Autodesk Fusion 360 part; units mm, degrees
(part 5 of 6)
  spline S1504 degree 3 poles (-29.6521, 8.8842) (-29.6849, 8.8897) (-29.7178, 8.8951) (-29.7517, 8.9007) knots 0 0 0 0 1 1 1 1
  spline S1505 degree 3 poles (-29.7517, 8.9007) (-30.0899, 8.9662) (-30.2987, 9.1721) (-30.5435, 9.4009) knots 0 0 0 0 1 1 1 1
  spline S1506 degree 3 poles (-30.5435, 9.4009) (-30.5714, 9.4268) (-30.5992, 9.4527) (-30.628, 9.4794) knots 0 0 0 0 1 1 1 1
  spline S1507 degree 3 poles (-30.628, 9.4794) (-30.6858, 9.5332) (-30.7436, 9.587) (-30.8013, 9.6409) knots 0 0 0 0 1 1 1 1
  spline S1508 degree 3 poles (-30.8013, 9.6409) (-30.8812, 9.7151) (-30.9615, 9.7888) (-31.0421, 9.8622) knots 0 0 0 0 1 1 1 1
  spline S1509 degree 3 poles (-31.0421, 9.8622) (-31.5525, 10.3296) (-31.9981, 10.8199) (-32.3801, 11.398) knots 0 0 0 0 1 1 1 1
  spline S1510 degree 3 poles (-32.3801, 11.398) (-32.528, 11.3037) (-32.625, 11.1724) (-32.732, 11.0364) knots 0 0 0 0 1 1 1 1
  spline S1511 degree 3 poles (-32.732, 11.0364) (-33.557, 10.0137) (-34.574, 9.1658) (-35.5651, 8.3103) knots 0 0 0 0 1 1 1 1
  spline S1512 degree 3 poles (-35.5651, 8.3103) (-36.1522, 7.8032) (-36.7179, 7.2786) (-37.2683, 6.7319) knots 0 0 0 0 1 1 1 1
  spline S1513 degree 3 poles (-37.2683, 6.7319) (-37.3268, 6.6738) (-37.3856, 6.6161) (-37.4451, 6.559) knots 0 0 0 0 1 1 1 1
  spline S1514 degree 3 poles (-37.4451, 6.559) (-37.6128, 6.3958) (-37.67, 6.2769) (-37.6736, 6.0447) knots 0 0 0 0 1 1 1 1
  spline S1515 degree 3 poles (-37.6736, 6.0447) (-37.6346, 5.5351) (-37.3928, 5.1499) (-37.0124, 4.8179) knots 0 0 0 0 1 1 1 1
  spline S1516 degree 3 poles (-37.0124, 4.8179) (-36.5513, 4.4276) (-36.5513, 4.4276) (-36.3386, 4.4) knots 0 0 0 0 1 1 1 1
  spline S1517 degree 3 poles (-36.3386, 4.4) (-36.3018, 4.395) (-36.265, 4.3899) (-36.227, 4.3848) knots 0 0 0 0 1 1 1 1
  spline S1518 degree 3 poles (-36.227, 4.3848) (-36.168, 4.377) (-36.168, 4.377) (-36.1079, 4.369) knots 0 0 0 0 1 1 1 1
  spline S1519 degree 3 poles (-36.1079, 4.369) (-35.784, 4.324) (-35.4699, 4.2678) (-35.153, 4.1868) knots 0 0 0 0 1 1 1 1
  spline S1520 degree 3 poles (-35.153, 4.1868) (-34.7861, 4.0991) (-34.7861, 4.0991) (-34.5906, 4.1538) knots 0 0 0 0 1 1 1 1
  spline S1521 degree 3 poles (-34.5906, 4.1538) (-34.562, 4.161) (-34.5334, 4.1682) (-34.504, 4.1757) knots 0 0 0 0 1 1 1 1
  spline S1522 degree 3 poles (-34.504, 4.1757) (-34.3447, 4.2643) (-34.2689, 4.4165) (-34.2111, 4.5847) knots 0 0 0 0 1 1 1 1
  spline S1523 degree 3 poles (-34.2111, 4.5847) (-34.2006, 4.6292) (-34.19, 4.6736) (-34.1792, 4.7194) knots 0 0 0 0 1 1 1 1
  spline S1524 degree 3 poles (-34.1792, 4.7194) (-34.1671, 4.7684) (-34.1549, 4.8174) (-34.1424, 4.8679) knots 0 0 0 0 1 1 1 1
  spline S1525 degree 3 poles (-34.1424, 4.8679) (-34.1181, 4.9703) (-34.0938, 5.0727) (-34.0695, 5.1751) knots 0 0 0 0 1 1 1 1
  spline S1526 degree 3 poles (-34.0695, 5.1751) (-34.0573, 5.2241) (-34.0452, 5.2731) (-34.0327, 5.3236) knots 0 0 0 0 1 1 1 1
  spline S1527 degree 3 poles (-34.0327, 5.3236) (-34.0222, 5.368) (-34.0116, 5.4125) (-34.0008, 5.4583) knots 0 0 0 0 1 1 1 1
  spline S1528 degree 3 poles (-34.0008, 5.4583) (-33.9132, 5.7136) (-33.7371, 5.8865) (-33.5439, 6.0655) knots 0 0 0 0 1 1 1 1
  spline S1529 degree 3 poles (-33.5439, 6.0655) (-33.5224, 6.0865) (-33.5008, 6.1074) (-33.4786, 6.129) knots 0 0 0 0 1 1 1 1
  spline S1530 degree 3 poles (-33.4786, 6.129) (-33.3655, 6.2415) (-33.3655, 6.2415) (-33.2182, 6.2846) knots 0 0 0 0 1 1 1 1
  spline S1531 degree 3 poles (-33.2182, 6.2846) (-33.0141, 6.247) (-32.8227, 6.1575) (-32.6303, 6.082) knots 0 0 0 0 1 1 1 1
  spline S1532 degree 3 poles (-32.6303, 6.082) (-32.5855, 6.0649) (-32.5407, 6.0479) (-32.4945, 6.0303) knots 0 0 0 0 1 1 1 1
  spline S1533 degree 3 poles (-32.4945, 6.0303) (-32.0082, 5.863) (-32.0082, 5.863) (-31.6692, 5.5102) knots 0 0 0 0 1 1 1 1
  spline S1534 degree 3 poles (-31.6692, 5.5102) (-31.6586, 5.4636) (-31.648, 5.417) (-31.6372, 5.369) knots 0 0 0 0 1 1 1 1
  spline S1535 degree 3 poles (-31.6372, 5.369) (-31.6008, 5.2148) (-31.5746, 5.1185) (-31.4738, 4.9954) knots 0 0 0 0 1 1 1 1
  spline S1536 degree 3 poles (-31.4738, 4.9954) (-31.2492, 4.8565) (-30.9935, 4.9477) (-30.7479, 4.9966) knots 0 0 0 0 1 1 1 1
  spline S1537 degree 3 poles (-30.7479, 4.9966) (-29.8977, 5.151) (-28.9911, 4.9807) (-28.217, 4.5961) knots 0 0 0 0 1 1 1 1
  spline S1538 degree 3 poles (-28.217, 4.5961) (-27.9097, 4.4451) (-27.5745, 4.3729) (-27.2439, 4.29) knots 0 0 0 0 1 1 1 1
  spline S1539 degree 3 poles (-27.2439, 4.29) (-27.2287, 4.0874) (-27.2198, 3.9243) (-27.3123, 3.741) knots 0 0 0 0 1 1 1 1
  spline S1540 degree 3 poles (-27.3123, 3.741) (-27.4452, 3.6719) (-27.5859, 3.6427) (-27.7313, 3.6097) knots 0 0 0 0 1 1 1 1
  spline S1541 degree 3 poles (-27.7313, 3.6097) (-27.7948, 3.5938) (-27.7948, 3.5938) (-27.8596, 3.5776) knots 0 0 0 0 1 1 1 1
  spline S1542 degree 3 poles (-27.8596, 3.5776) (-27.9954, 3.5438) (-28.1316, 3.5116) (-28.2679, 3.4795) knots 0 0 0 0 1 1 1 1
  spline S1543 degree 3 poles (-28.2679, 3.4795) (-28.4456, 3.4363) (-28.6231, 3.3925) (-28.8006, 3.3488) knots 0 0 0 0 1 1 1 1
  spline S1544 degree 3 poles (-28.8006, 3.3488) (-28.8433, 3.3384) (-28.886, 3.3279) (-28.93, 3.3172) knots 0 0 0 0 1 1 1 1
  spline S1545 degree 3 poles (-28.93, 3.3172) (-29.6689, 3.1354) (-30.0673, 2.971) (-30.4724, 2.3083) knots 0 0 0 0 1 1 1 1
  spline S1546 degree 3 poles (-30.4724, 2.3083) (-30.5322, 2.206) (-30.5883, 2.1042) (-30.64, 1.9976) knots 0 0 0 0 1 1 1 1
  spline S1547 degree 3 poles (-30.64, 1.9976) (-30.5984, 2.0078) (-30.5568, 2.018) (-30.5139, 2.0286) knots 0 0 0 0 1 1 1 1
  spline S1548 degree 3 poles (-30.5139, 2.0286) (-30.4575, 2.0408) (-30.4011, 2.053) (-30.3446, 2.0652) knots 0 0 0 0 1 1 1 1
  spline S1549 degree 3 poles (-30.3446, 2.0652) (-30.3174, 2.0721) (-30.2903, 2.0789) (-30.2622, 2.086) knots 0 0 0 0 1 1 1 1
  spline S1550 degree 3 poles (-30.2622, 2.086) (-30.0393, 2.1318) (-29.9052, 2.0843) (-29.7037, 1.9852) knots 0 0 0 0 1 1 1 1
  spline S1551 degree 3 poles (-29.7037, 1.9852) (-29.5915, 1.9317) (-29.4796, 1.8907) (-29.362, 1.8509) knots 0 0 0 0 1 1 1 1
  spline S1552 degree 3 poles (-29.362, 1.8509) (-29.3215, 1.8371) (-29.2809, 1.8234) (-29.2392, 1.8092) knots 0 0 0 0 1 1 1 1
  spline S1553 degree 3 poles (-29.2392, 1.8092) (-29.1763, 1.7879) (-29.1763, 1.7879) (-29.1121, 1.7662) knots 0 0 0 0 1 1 1 1
  spline S1554 degree 3 poles (-29.1121, 1.7662) (-28.5135, 1.5583) (-27.953, 1.3163) (-27.4238, 0.9662) knots 0 0 0 0 1 1 1 1
  spline S1555 degree 3 poles (-27.4238, 0.9662) (-27.3036, 0.8907) (-27.1824, 0.829) (-27.0541, 0.7685) knots 0 0 0 0 1 1 1 1
  spline S1556 degree 3 poles (-27.0541, 0.7685) (-26.5687, 0.5436) (-26.5687, 0.5436) (-26.1888, 0.1801) knots 0 0 0 0 1 1 1 1
  spline S1557 degree 3 poles (-26.1888, 0.1801) (-26.1759, 0.1353) (-26.163, 0.0906) (-26.1497, 0.0444) knots 0 0 0 0 1 1 1 1
  spline S1558 degree 3 poles (-26.1497, 0.0444) (-26.0853, -0.1312) (-26.0071, -0.1838) (-25.8533, -0.2874) knots 0 0 0 0 1 1 1 1
  spline S1559 degree 3 poles (-25.8533, -0.2874) (-25.7876, -0.333) (-25.7876, -0.333) (-25.7206, -0.3795) knots 0 0 0 0 1 1 1 1
  spline S1560 degree 3 poles (-25.7206, -0.3795) (-25.5423, -0.4774) (-25.382, -0.5513) (-25.1755, -0.5023) knots 0 0 0 0 1 1 1 1
  spline S1561 degree 3 poles (-25.1755, -0.5023) (-25.0762, -0.446) (-24.9885, -0.3833) (-24.8988, -0.3127) knots 0 0 0 0 1 1 1 1
  spline S1562 degree 3 poles (-24.8988, -0.3127) (-24.7642, -0.2053) (-24.7642, -0.2053) (-24.6005, -0.1594) knots 0 0 0 0 1 1 1 1
  spline S1563 degree 3 poles (-24.6005, -0.1594) (-24.6093, -0.1305) (-24.6181, -0.1015) (-24.6271, -0.0716) knots 0 0 0 0 1 1 1 1
  spline S1564 degree 3 poles (-24.6271, -0.0716) (-24.6467, 0.0436) (-24.6467, 0.0436) (-24.579, 0.1405) knots 0 0 0 0 1 1 1 1
  spline S1565 degree 3 poles (-24.579, 0.1405) (-24.5505, 0.173) (-24.522, 0.2056) (-24.4927, 0.2391) knots 0 0 0 0 1 1 1 1
  spline S1566 degree 3 poles (-24.4927, 0.2391) (-24.4517, 0.2881) (-24.4517, 0.2881) (-24.4099, 0.3381) knots 0 0 0 0 1 1 1 1
  spline S1567 degree 3 poles (-24.4099, 0.3381) (-24.0952, 0.5882) (-23.6684, 0.6419) (-23.2824, 0.7107) knots 0 0 0 0 1 1 1 1
  spline S1568 degree 3 poles (-23.2824, 0.7107) (-23.2555, 0.7155) (-23.2286, 0.7203) (-23.2009, 0.7253) knots 0 0 0 0 1 1 1 1
  spline S1569 degree 3 poles (-23.2009, 0.7253) (-22.6594, 0.8201) (-22.134, 0.8278) (-21.5864, 0.7851) knots 0 0 0 0 1 1 1 1
  spline S1570 degree 3 poles (-21.5864, 0.7851) (-21.5162, 0.78) (-21.5162, 0.78) (-21.4446, 0.7748) knots 0 0 0 0 1 1 1 1
  spline S1571 degree 3 poles (-21.4446, 0.7748) (-21.0146, 0.7409) (-20.5888, 0.6847) (-20.1617, 0.6259) knots 0 0 0 0 1 1 1 1
  spline S1572 degree 3 poles (-20.1617, 0.6259) (-19.7246, 0.5657) (-19.2882, 0.5102) (-18.8488, 0.47) knots 0 0 0 0 1 1 1 1
  spline S1573 degree 3 poles (-18.8488, 0.47) (-18.6938, 0.4557) (-18.5402, 0.4394) (-18.3863, 0.4148) knots 0 0 0 0 1 1 1 1
  spline S1574 degree 3 poles (-18.3863, 0.4148) (-18.1653, 0.3795) (-17.9433, 0.3654) (-17.7201, 0.3516) knots 0 0 0 0 1 1 1 1
  spline S1575 degree 3 poles (-17.7201, 0.3516) (-17.6747, 0.3487) (-17.6293, 0.3458) (-17.5825, 0.3428) knots 0 0 0 0 1 1 1 1
  spline S1576 degree 3 poles (-17.5825, 0.3428) (-17.286, 0.3259) (-16.9952, 0.3274) (-16.6988, 0.3432) knots 0 0 0 0 1 1 1 1
  spline S1577 degree 3 poles (-16.6988, 0.3432) (-16.4354, 0.3568) (-16.2244, 0.3521) (-15.9742, 0.2575) knots 0 0 0 0 1 1 1 1
  spline S1578 degree 3 poles (-15.9742, 0.2575) (-15.5032, 0.1043) (-15.0149, 0.1628) (-14.5414, 0.2581) knots 0 0 0 0 1 1 1 1
  spline S1579 degree 3 poles (-14.5414, 0.2581) (-13.6214, 0.4402) (-12.5735, 0.5414) (-11.6609, 0.2614) knots 0 0 0 0 1 1 1 1
  spline S1580 degree 3 poles (-11.6609, 0.2614) (-11.3698, 0.1728) (-11.1253, 0.2064) (-10.828, 0.2553) knots 0 0 0 0 1 1 1 1
  spline S1581 degree 3 poles (-10.828, 0.2553) (-10.7752, 0.2636) (-10.7223, 0.2718) (-10.6678, 0.2803) knots 0 0 0 0 1 1 1 1
  spline S1582 degree 3 poles (-10.6678, 0.2803) (-10.5167, 0.3041) (-10.3657, 0.3292) (-10.2148, 0.3543) knots 0 0 0 0 1 1 1 1
  spline S1583 degree 3 poles (-10.2148, 0.3543) (-10.1066, 0.3721) (-9.9983, 0.3894) (-9.8901, 0.4065) knots 0 0 0 0 1 1 1 1
  spline S1584 degree 3 poles (-9.8901, 0.4065) (-7.4812, 0.7887) (-7.4812, 0.7887) (-6.9237, 1.3531) knots 0 0 0 0 1 1 1 1
  spline S1585 degree 3 poles (-6.9237, 1.3531) (-6.5081, 1.772) (-5.7865, 1.7818) (-5.232, 1.7842) knots 0 0 0 0 1 1 1 1
  spline S1586 degree 3 poles (-5.232, 1.7842) (-4.8504, 1.7821) (-4.4705, 1.759) (-4.0903, 1.7266) knots 0 0 0 0 1 1 1 1
  spline S1587 degree 3 poles (-4.0903, 1.7266) (-3.602, 1.6859) (-3.1526, 1.705) (-2.6732, 1.8089) knots 0 0 0 0 1 1 1 1
  spline S1588 degree 3 poles (-2.6732, 1.8089) (-2.464, 1.8442) (-2.464, 1.8442) (-2.2713, 1.7712) knots 0 0 0 0 1 1 1 1
  spline S1589 degree 3 poles (-2.2713, 1.7712) (-2.0081, 1.5146) (-1.8399, 1.165) (-1.6596, 0.8488) knots 0 0 0 0 1 1 1 1
  spline S1590 degree 3 poles (-1.6596, 0.8488) (-1.5014, 0.5801) (-1.3373, 0.3693) (-1.1063, 0.1596) knots 0 0 0 0 1 1 1 1
  spline S1591 degree 3 poles (-1.1063, 0.1596) (-0.9857, 0.0491) (-0.8826, -0.0712) (-0.7801, -0.1984) knots 0 0 0 0 1 1 1 1
  spline S1592 degree 3 poles (-0.7801, -0.1984) (-0.7529, -0.2314) (-0.7529, -0.2314) (-0.7251, -0.265) knots 0 0 0 0 1 1 1 1
  spline S1593 degree 3 poles (-0.7251, -0.265) (-0.6378, -0.3574) (-0.6378, -0.3574) (-0.5878, -0.4691) knots 0 0 0 0 1 1 1 1
  spline S1594 degree 3 poles (-0.5878, -0.4691) (-1.0381, -0.5386) (-1.4685, -0.5208) (-1.9212, -0.4926) knots 0 0 0 0 1 1 1 1
  spline S1595 degree 3 poles (-1.9212, -0.4926) (-2.6362, -0.4486) (-3.3429, -0.4263) (-4.0589, -0.4615) knots 0 0 0 0 1 1 1 1
  spline S1596 degree 3 poles (-4.0589, -0.4615) (-4.1392, -0.464) (-4.1392, -0.464) (-4.221, -0.4666) knots 0 0 0 0 1 1 1 1
  spline S1597 degree 3 poles (-4.221, -0.4666) (-4.3917, -0.4753) (-4.5589, -0.5022) (-4.7277, -0.5283) knots 0 0 0 0 1 1 1 1
  spline S1598 degree 3 poles (-4.7277, -0.5283) (-5.2586, -0.6093) (-5.7689, -0.6274) (-6.3047, -0.6097) knots 0 0 0 0 1 1 1 1
  spline S1599 degree 3 poles (-6.3047, -0.6097) (-7.0546, -0.5862) (-7.7994, -0.62) (-8.5483, -0.657) knots 0 0 0 0 1 1 1 1
  spline S1600 degree 3 poles (-8.5483, -0.657) (-8.711, -0.665) (-8.8738, -0.6721) (-9.0367, -0.679) knots 0 0 0 0 1 1 1 1
  spline S1601 degree 3 poles (-9.0367, -0.679) (-9.123, -0.6828) (-9.2093, -0.6866) (-9.2956, -0.6904) knots 0 0 0 0 1 1 1 1
  spline S1602 degree 3 poles (-9.2956, -0.6904) (-9.333, -0.6919) (-9.3705, -0.6934) (-9.4091, -0.695) knots 0 0 0 0 1 1 1 1
  spline S1603 degree 3 poles (-9.4091, -0.695) (-9.7302, -0.7101) (-10.0266, -0.7252) (-10.3014, -0.9013) knots 0 0 0 0 1 1 1 1
  spline S1604 degree 3 poles (-10.3014, -0.9013) (-10.4201, -0.9361) (-10.5404, -0.9572) (-10.6622, -0.9779) knots 0 0 0 0 1 1 1 1
  spline S1605 degree 3 poles (-10.6622, -0.9779) (-10.6975, -0.9841) (-10.7328, -0.9902) (-10.7692, -0.9966) knots 0 0 0 0 1 1 1 1
  spline S1606 degree 3 poles (-10.7692, -0.9966) (-11.0516, -1.0422) (-11.3271, -1.052) (-11.6127, -1.0531) knots 0 0 0 0 1 1 1 1
  spline S1607 degree 3 poles (-11.6127, -1.0531) (-12.0092, -1.0582) (-12.4812, -1.0899) (-12.8497, -1.2478) knots 0 0 0 0 1 1 1 1
  spline S1608 degree 3 poles (-12.8497, -1.2478) (-13.0113, -1.3061) (-13.1766, -1.3299) (-13.3458, -1.3581) knots 0 0 0 0 1 1 1 1
  spline S1609 degree 3 poles (-13.3458, -1.3581) (-13.425, -1.3717) (-13.5041, -1.3853) (-13.5833, -1.3989) knots 0 0 0 0 1 1 1 1
  spline S1610 degree 3 poles (-13.5833, -1.3989) (-13.6249, -1.406) (-13.6664, -1.4131) (-13.7093, -1.4204) knots 0 0 0 0 1 1 1 1
  spline S1611 degree 3 poles (-13.7093, -1.4204) (-14.6093, -1.574) (-15.5055, -1.7412) (-16.3978, -1.935) knots 0 0 0 0 1 1 1 1
  spline S1612 degree 3 poles (-16.3978, -1.935) (-16.4275, -1.9414) (-16.4572, -1.9479) (-16.4878, -1.9545) knots 0 0 0 0 1 1 1 1
  spline S1613 degree 3 poles (-16.4878, -1.9545) (-18.156, -2.318) (-19.8004, -2.7903) (-21.3671, -3.4747) knots 0 0 0 0 1 1 1 1
  spline S1614 degree 3 poles (-21.3671, -3.4747) (-21.4063, -3.4915) (-21.4063, -3.4915) (-21.4462, -3.5087) knots 0 0 0 0 1 1 1 1
  spline S1615 degree 3 poles (-21.4462, -3.5087) (-22.0107, -3.7526) (-22.0107, -3.7526) (-22.1548, -4.0744) knots 0 0 0 0 1 1 1 1
  spline S1616 degree 3 poles (-22.1548, -4.0744) (-22.207, -4.2706) (-22.2494, -4.4648) (-22.2829, -4.665) knots 0 0 0 0 1 1 1 1
  spline S1617 degree 3 poles (-22.2829, -4.665) (-22.3455, -4.9895) (-22.4619, -5.2838) (-22.5875, -5.5875) knots 0 0 0 0 1 1 1 1
  spline S1618 degree 3 poles (-22.5875, -5.5875) (-22.8538, -6.2352) (-23.0714, -6.8218) (-22.9351, -7.5256) knots 0 0 0 0 1 1 1 1
  spline S1619 degree 3 poles (-22.9351, -7.5256) (-22.9208, -7.601) (-22.9066, -7.6763) (-22.8925, -7.7516) knots 0 0 0 0 1 1 1 1
  spline S1620 degree 3 poles (-22.8925, -7.7516) (-22.8855, -7.7887) (-22.8785, -7.8257) (-22.8713, -7.8639) knots 0 0 0 0 1 1 1 1
  spline S1621 degree 3 poles (-22.8713, -7.8639) (-22.8661, -7.8916) (-22.8608, -7.9193) (-22.8555, -7.9479) knots 0 0 0 0 1 1 1 1
  spline S1622 degree 3 poles (-22.8555, -7.9479) (-22.8275, -7.9418) (-22.7995, -7.9358) (-22.7707, -7.9295) knots 0 0 0 0 1 1 1 1
  spline S1623 degree 3 poles (-22.7707, -7.9295) (-21.9127, -7.7443) (-21.0517, -7.577) (-20.1891, -7.4145) knots 0 0 0 0 1 1 1 1
  spline S1624 degree 3 poles (-20.1891, -7.4145) (-20.0161, -7.3818) (-19.8432, -7.3491) (-19.6703, -7.3163) knots 0 0 0 0 1 1 1 1
  spline S1625 degree 3 poles (-19.6703, -7.3163) (-19.3346, -7.2528) (-18.9989, -7.1894) (-18.6631, -7.1261) knots 0 0 0 0 1 1 1 1
  spline S1626 degree 3 poles (-18.6631, -7.1261) (-18.6798, -7.047) (-18.6964, -6.9679) (-18.713, -6.8888) knots 0 0 0 0 1 1 1 1
  spline S1627 degree 3 poles (-18.713, -6.8888) (-18.7272, -6.7939) (-18.7272, -6.7939) (-18.6607, -6.6713) knots 0 0 0 0 1 1 1 1
  spline S1628 degree 3 poles (-18.6607, -6.6713) (-18.6019, -6.7799) (-18.5832, -6.8517) (-18.5638, -6.9717) knots 0 0 0 0 1 1 1 1
  spline S1629 degree 3 poles (-18.5638, -6.9717) (-18.5558, -7.0204) (-18.5558, -7.0204) (-18.5476, -7.07) knots 0 0 0 0 1 1 1 1
  spline S1630 degree 3 poles (-18.5476, -7.07) (-18.5437, -7.0948) (-18.5399, -7.1195) (-18.5359, -7.1449) knots 0 0 0 0 1 1 1 1
  spline S1631 degree 3 poles (-18.5359, -7.1449) (-17.7698, -7.0108) (-17.0038, -6.8765) (-16.2378, -6.7419) knots 0 0 0 0 1 1 1 1
  spline S1632 degree 3 poles (-16.2378, -6.7419) (-15.882, -6.6793) (-15.5262, -6.6169) (-15.1703, -6.5546) knots 0 0 0 0 1 1 1 1
  spline S1633 degree 3 poles (-15.1703, -6.5546) (-14.8594, -6.5002) (-14.5486, -6.4457) (-14.2378, -6.3909) knots 0 0 0 0 1 1 1 1
  spline S1634 degree 3 poles (-14.2378, -6.3909) (-14.0738, -6.3621) (-13.9099, -6.3333) (-13.7459, -6.3047) knots 0 0 0 0 1 1 1 1
  spline S1635 degree 3 poles (-13.7459, -6.3047) (-13.0353, -6.1807) (-12.3271, -6.0499) (-11.6216, -5.8989) knots 0 0 0 0 1 1 1 1
  spline S1636 degree 3 poles (-11.6216, -5.8989) (-11.2592, -5.8216) (-10.8959, -5.7543) (-10.5306, -5.6921) knots 0 0 0 0 1 1 1 1
  spline S1637 degree 3 poles (-10.5306, -5.6921) (-10.537, -5.6681) (-10.5434, -5.6441) (-10.5499, -5.6193) knots 0 0 0 0 1 1 1 1
  spline S1638 degree 3 poles (-10.5499, -5.6193) (-10.6239, -5.3254) (-10.546, -5.1439) (-10.4003, -4.8876) knots 0 0 0 0 1 1 1 1
  spline S1639 degree 3 poles (-10.4003, -4.8876) (-10.2186, -4.5663) (-10.1227, -4.2298) (-10.0202, -3.877) knots 0 0 0 0 1 1 1 1
  spline S1640 degree 3 poles (-10.0202, -3.877) (-9.888, -3.4365) (-9.7021, -2.9191) (-9.2883, -2.6642) knots 0 0 0 0 1 1 1 1
  spline S1641 degree 3 poles (-9.2883, -2.6642) (-9.2006, -2.6368) (-9.1117, -2.6128) (-9.0223, -2.5914) knots 0 0 0 0 1 1 1 1
  spline S1642 degree 3 poles (-9.0223, -2.5914) (-8.976, -2.5802) (-8.9296, -2.5689) (-8.8818, -2.5573) knots 0 0 0 0 1 1 1 1
  spline S1643 degree 3 poles (-8.8818, -2.5573) (-8.8464, -2.549) (-8.8111, -2.5408) (-8.7746, -2.5323) knots 0 0 0 0 1 1 1 1
  spline S1644 degree 3 poles (-8.7746, -2.5323) (-8.6277, -2.9907) (-8.9453, -3.4949) (-9.1361, -3.9008) knots 0 0 0 0 1 1 1 1
  spline S1645 degree 3 poles (-9.1361, -3.9008) (-9.1527, -3.9363) (-9.1693, -3.9717) (-9.1864, -4.0082) knots 0 0 0 0 1 1 1 1
  spline S1646 degree 3 poles (-9.1864, -4.0082) (-9.2015, -4.0399) (-9.2166, -4.0717) (-9.2322, -4.1044) knots 0 0 0 0 1 1 1 1
  spline S1647 degree 3 poles (-9.2322, -4.1044) (-9.2944, -4.2539) (-9.2823, -4.3662) (-9.2541, -4.5213) knots 0 0 0 0 1 1 1 1
  spline S1648 degree 3 poles (-9.2541, -4.5213) (-9.2434, -4.5803) (-9.2434, -4.5803) (-9.2326, -4.6405) knots 0 0 0 0 1 1 1 1
  spline S1649 degree 3 poles (-9.2326, -4.6405) (-9.225, -4.6815) (-9.2175, -4.7225) (-9.2097, -4.7647) knots 0 0 0 0 1 1 1 1
  spline S1650 degree 3 poles (-9.2097, -4.7647) (-9.2022, -4.8062) (-9.1947, -4.8476) (-9.187, -4.8903) knots 0 0 0 0 1 1 1 1
  spline S1651 degree 3 poles (-9.187, -4.8903) (-9.1684, -4.9927) (-9.1497, -5.0951) (-9.1308, -5.1974) knots 0 0 0 0 1 1 1 1
  spline S1652 degree 3 poles (-9.1308, -5.1974) (-8.1927, -5.0811) (-8.1927, -5.0811) (-7.9563, -4.8201) knots 0 0 0 0 1 1 1 1
  spline S1653 degree 3 poles (-7.9563, -4.8201) (-7.9348, -4.7907) (-7.9134, -4.7613) (-7.8912, -4.731) knots 0 0 0 0 1 1 1 1
  spline S1654 degree 3 poles (-7.8912, -4.731) (-7.8677, -4.7008) (-7.8442, -4.6706) (-7.82, -4.6395) knots 0 0 0 0 1 1 1 1
  spline S1655 degree 3 poles (-7.82, -4.6395) (-7.5084, -4.191) (-7.4309, -3.6293) (-7.3384, -3.1024) knots 0 0 0 0 1 1 1 1
  spline S1656 degree 3 poles (-7.3384, -3.1024) (-7.3284, -3.0467) (-7.3284, -3.0467) (-7.3183, -2.99) knots 0 0 0 0 1 1 1 1
  spline S1657 degree 3 poles (-7.3183, -2.99) (-7.3098, -2.9401) (-7.3098, -2.9401) (-7.301, -2.8893) knots 0 0 0 0 1 1 1 1
  spline S1658 degree 3 poles (-7.301, -2.8893) (-7.2843, -2.7989) (-7.2843, -2.7989) (-7.2146, -2.7116) knots 0 0 0 0 1 1 1 1
  spline S1659 degree 3 poles (-7.2146, -2.7116) (-7.0441, -2.6485) (-6.9505, -2.6356) (-6.7773, -2.6953) knots 0 0 0 0 1 1 1 1
  spline S1660 degree 3 poles (-6.7773, -2.6953) (-6.2734, -2.9329) (-5.8702, -3.2655) (-5.4833, -3.6606) knots 0 0 0 0 1 1 1 1
  spline S1661 degree 3 poles (-5.4833, -3.6606) (-5.4357, -3.7085) (-5.3853, -3.7537) (-5.3343, -3.798) knots 0 0 0 0 1 1 1 1
  spline S1662 degree 3 poles (-5.3343, -3.798) (-5.1537, -4.0794) (-5.2499, -4.4937) (-5.291, -4.8069) knots 0 0 0 0 1 1 1 1
  spline S1663 degree 3 poles (-5.291, -4.8069) (-5.3004, -4.879) (-5.3004, -4.879) (-5.3099, -4.9525) knots 0 0 0 0 1 1 1 1
  spline S1664 degree 3 poles (-5.3099, -4.9525) (-5.4375, -5.8796) (-5.6805, -6.7775) (-5.9228, -7.6795) knots 0 0 0 0 1 1 1 1
  spline S1665 degree 3 poles (-5.9228, -7.6795) (-6.341, -9.2373) (-6.694, -10.7765) (-6.6192, -12.3989) knots 0 0 0 0 1 1 1 1
  spline S1666 degree 3 poles (-6.6192, -12.3989) (-6.5997, -13.1562) (-7.0156, -13.7676) (-7.4367, -14.3614) knots 0 0 0 0 1 1 1 1
  spline S1667 degree 3 poles (-7.4367, -14.3614) (-7.5397, -14.5105) (-7.6316, -14.6652) (-7.7229, -14.8216) knots 0 0 0 0 1 1 1 1
  spline S1668 degree 3 poles (-7.7229, -14.8216) (-7.7457, -14.8591) (-7.7685, -14.8966) (-7.792, -14.9352) knots 0 0 0 0 1 1 1 1
  spline S1669 degree 3 poles (-7.792, -14.9352) (-8.1036, -15.4636) (-8.2571, -15.9713) (-8.3217, -16.5794) knots 0 0 0 0 1 1 1 1
  spline S1670 degree 3 poles (-8.3217, -16.5794) (-8.3253, -16.6117) (-8.3288, -16.644) (-8.3325, -16.6773) knots 0 0 0 0 1 1 1 1
  spline S1671 degree 3 poles (-8.3325, -16.6773) (-8.3523, -16.8594) (-8.3712, -17.0416) (-8.3895, -17.2239) knots 0 0 0 0 1 1 1 1
  spline S1672 degree 3 poles (-8.3895, -17.2239) (-8.4151, -17.4784) (-8.443, -17.7327) (-8.4711, -17.987) knots 0 0 0 0 1 1 1 1
  spline S1673 degree 3 poles (-8.4711, -17.987) (-8.5492, -18.6956) (-8.6202, -19.4047) (-8.6899, -20.1141) knots 0 0 0 0 1 1 1 1
  spline S1674 degree 3 poles (-8.6899, -20.1141) (-8.798, -20.1185) (-8.8448, -20.1125) (-8.9297, -20.0427) knots 0 0 0 0 1 1 1 1
  spline S1675 degree 3 poles (-8.9297, -20.0427) (-8.9539, -20.0155) (-8.9781, -19.9882) (-9.0031, -19.9601) knots 0 0 0 0 1 1 1 1
  spline S1676 degree 3 poles (-9.0031, -19.9601) (-9.0309, -19.9292) (-9.0588, -19.8983) (-9.0875, -19.8665) knots 0 0 0 0 1 1 1 1
  spline S1677 degree 3 poles (-9.0875, -19.8665) (-9.1172, -19.8326) (-9.147, -19.7987) (-9.1776, -19.7638) knots 0 0 0 0 1 1 1 1
  spline S1678 degree 3 poles (-9.1776, -19.7638) (-9.2086, -19.7292) (-9.2397, -19.6946) (-9.2717, -19.6589) knots 0 0 0 0 1 1 1 1
  spline S1679 degree 3 poles (-9.2717, -19.6589) (-9.3726, -19.5462) (-9.473, -19.4331) (-9.5734, -19.3199) knots 0 0 0 0 1 1 1 1
  spline S1680 degree 3 poles (-9.5734, -19.3199) (-9.6786, -19.2022) (-9.784, -19.0847) (-9.8894, -18.9673) knots 0 0 0 0 1 1 1 1
  spline S1681 degree 3 poles (-9.8894, -18.9673) (-9.9561, -18.893) (-10.0227, -18.8186) (-10.0891, -18.7441) knots 0 0 0 0 1 1 1 1
  spline S1682 degree 3 poles (-10.0891, -18.7441) (-10.1195, -18.71) (-10.15, -18.6759) (-10.1814, -18.6408) knots 0 0 0 0 1 1 1 1
  spline S1683 degree 3 poles (-10.1814, -18.6408) (-10.2081, -18.6108) (-10.2348, -18.5809) (-10.2623, -18.55) knots 0 0 0 0 1 1 1 1
  spline S1684 degree 3 poles (-10.2623, -18.55) (-10.5301, -18.2688) (-10.5301, -18.2688) (-10.7539, -18.2475) knots 0 0 0 0 1 1 1 1
  spline S1685 degree 3 poles (-10.7539, -18.2475) (-11.0414, -18.2599) (-11.2582, -18.344) (-11.4931, -18.5069) knots 0 0 0 0 1 1 1 1
  spline S1686 degree 3 poles (-11.4931, -18.5069) (-11.5637, -18.561) (-11.5637, -18.561) (-11.647, -18.5702) knots 0 0 0 0 1 1 1 1
  spline S1687 degree 3 poles (-11.647, -18.5702) (-11.662, -18.6417) (-11.6769, -18.7132) (-11.6919, -18.7847) knots 0 0 0 0 1 1 1 1
  spline S1688 degree 3 poles (-11.6919, -18.7847) (-11.7016, -18.8162) (-11.7114, -18.8477) (-11.7215, -18.8802) knots 0 0 0 0 1 1 1 1
  spline S1689 degree 3 poles (-11.7215, -18.8802) (-11.7744, -19.2944) (-11.5857, -19.7618) (-11.3548, -20.0961) knots 0 0 0 0 1 1 1 1
  spline S1690 degree 3 poles (-11.3548, -20.0961) (-11.1799, -20.3194) (-10.9429, -20.5448) (-10.6647, -20.6276) knots 0 0 0 0 1 1 1 1
  spline S1691 degree 3 poles (-10.6647, -20.6276) (-10.6662, -20.696) (-10.6678, -20.7644) (-10.6694, -20.835) knots 0 0 0 0 1 1 1 1
  spline S1692 degree 3 poles (-10.6694, -20.835) (-11.3822, -20.9275) (-12.0612, -20.3827) (-12.5969, -19.9769) knots 0 0 0 0 1 1 1 1
  spline S1693 degree 3 poles (-12.5969, -19.9769) (-12.706, -19.8868) (-12.812, -19.7941) (-12.9178, -19.7001) knots 0 0 0 0 1 1 1 1
  spline S1694 degree 3 poles (-12.9178, -19.7001) (-13.0662, -19.5733) (-13.2201, -19.4549) (-13.3758, -19.3372) knots 0 0 0 0 1 1 1 1
  spline S1695 degree 3 poles (-13.3758, -19.3372) (-13.4169, -19.3058) (-13.4169, -19.3058) (-13.4588, -19.2739) knots 0 0 0 0 1 1 1 1
  spline S1696 degree 3 poles (-13.4588, -19.2739) (-13.539, -19.2138) (-13.62, -19.1554) (-13.702, -19.0978) knots 0 0 0 0 1 1 1 1
  spline S1697 degree 3 poles (-13.702, -19.0978) (-13.7266, -19.0801) (-13.7512, -19.0625) (-13.7765, -19.0443) knots 0 0 0 0 1 1 1 1
  spline S1698 degree 3 poles (-13.7765, -19.0443) (-14.01, -18.8903) (-14.2547, -18.8454) (-14.527, -18.7966) knots 0 0 0 0 1 1 1 1
  spline S1699 degree 3 poles (-14.527, -18.7966) (-14.5711, -18.7881) (-14.6153, -18.7797) (-14.6607, -18.7709) knots 0 0 0 0 1 1 1 1
  spline S1700 degree 3 poles (-14.6607, -18.7709) (-15.1075, -18.6863) (-15.4557, -18.6668) (-15.851, -18.9247) knots 0 0 0 0 1 1 1 1
  spline S1701 degree 3 poles (-15.851, -18.9247) (-15.91, -18.9914) (-15.91, -18.9914) (-15.9238, -19.0833) knots 0 0 0 0 1 1 1 1
  spline S1702 degree 3 poles (-15.9238, -19.0833) (-15.8908, -19.5038) (-15.8376, -19.8736) (-15.5709, -20.2122) knots 0 0 0 0 1 1 1 1
  spline S1703 degree 3 poles (-15.5709, -20.2122) (-15.5404, -20.2536) (-15.5404, -20.2536) (-15.5093, -20.2959) knots 0 0 0 0 1 1 1 1
  spline S1704 degree 3 poles (-15.5093, -20.2959) (-15.2744, -20.6028) (-14.9762, -20.8389) (-14.679, -21.0824) knots 0 0 0 0 1 1 1 1
  spline S1705 degree 3 poles (-14.679, -21.0824) (-14.6543, -21.1027) (-14.6295, -21.1231) (-14.604, -21.144) knots 0 0 0 0 1 1 1 1
  spline S1706 degree 3 poles (-14.604, -21.144) (-14.4029, -21.3089) (-14.4029, -21.3089) (-14.3149, -21.3796) knots 0 0 0 0 1 1 1 1
  spline S1707 degree 3 poles (-14.3149, -21.3796) (-14.253, -21.4294) (-14.1916, -21.4799) (-14.1302, -21.5304) knots 0 0 0 0 1 1 1 1
  spline S1708 degree 3 poles (-14.1302, -21.5304) (-14.0951, -21.5588) (-14.0601, -21.5871) (-14.024, -21.6164) knots 0 0 0 0 1 1 1 1
  spline S1709 degree 3 poles (-14.024, -21.6164) (-13.9329, -21.7149) (-13.909, -21.7682) (-13.9098, -21.902) knots 0 0 0 0 1 1 1 1
  spline S1710 degree 3 poles (-13.9098, -21.902) (-14.003, -22.0122) (-14.003, -22.0122) (-14.1111, -22.0117) knots 0 0 0 0 1 1 1 1
  spline S1711 degree 3 poles (-14.1111, -22.0117) (-14.2358, -21.9971) (-14.344, -21.9673) (-14.4629, -21.9273) knots 0 0 0 0 1 1 1 1
  spline S1712 degree 3 poles (-14.4629, -21.9273) (-14.5032, -21.9141) (-14.5434, -21.901) (-14.5849, -21.8874) knots 0 0 0 0 1 1 1 1
  spline S1713 degree 3 poles (-14.5849, -21.8874) (-14.8141, -21.7901) (-14.9903, -21.6323) (-15.1762, -21.4696) knots 0 0 0 0 1 1 1 1
  spline S1714 degree 3 poles (-15.1762, -21.4696) (-15.3728, -21.3012) (-15.5695, -21.1598) (-15.7972, -21.0369) knots 0 0 0 0 1 1 1 1
  spline S1715 degree 3 poles (-15.7972, -21.0369) (-15.8322, -21.0179) (-15.8322, -21.0179) (-15.8679, -20.9986) knots 0 0 0 0 1 1 1 1
  spline S1716 degree 3 poles (-15.8679, -20.9986) (-16.0566, -20.8964) (-16.2462, -20.7957) (-16.4358, -20.6951) knots 0 0 0 0 1 1 1 1
  spline S1717 degree 3 poles (-16.4358, -20.6951) (-16.7511, -20.5273) (-17.0573, -20.3497) (-17.3571, -20.1554) knots 0 0 0 0 1 1 1 1
  spline S1718 degree 3 poles (-17.3571, -20.1554) (-17.3908, -20.1336) (-17.4246, -20.1119) (-17.4594, -20.0895) knots 0 0 0 0 1 1 1 1
  spline S1719 degree 3 poles (-17.4594, -20.0895) (-17.7732, -19.8796) (-18.0137, -19.6392) (-18.2019, -19.3107) knots 0 0 0 0 1 1 1 1
  spline S1720 degree 3 poles (-18.2019, -19.3107) (-18.287, -19.2116) (-18.3572, -19.1884) (-18.4833, -19.156) knots 0 0 0 0 1 1 1 1
  spline S1721 degree 3 poles (-18.4833, -19.156) (-18.6292, -19.1606) (-18.6292, -19.1606) (-18.7812, -19.1801) knots 0 0 0 0 1 1 1 1
  spline S1722 degree 3 poles (-18.7812, -19.1801) (-18.8319, -19.1864) (-18.8826, -19.1926) (-18.9348, -19.199) knots 0 0 0 0 1 1 1 1
  spline S1723 degree 3 poles (-18.9348, -19.199) (-18.9733, -19.2042) (-19.0117, -19.2095) (-19.0513, -19.2149) knots 0 0 0 0 1 1 1 1
  spline S1724 degree 3 poles (-19.0513, -19.2149) (-19.034, -19.2646) (-19.0167, -19.3144) (-18.9989, -19.3657) knots 0 0 0 0 1 1 1 1
  spline S1725 degree 3 poles (-18.9989, -19.3657) (-18.9237, -19.6243) (-18.9208, -19.8645) (-18.9997, -20.1223) knots 0 0 0 0 1 1 1 1
  spline S1726 degree 3 poles (-18.9997, -20.1223) (-19.1792, -20.4309) (-19.4037, -20.6478) (-19.6835, -20.8681) knots 0 0 0 0 1 1 1 1
  spline S1727 degree 3 poles (-19.6835, -20.8681) (-19.7783, -20.9548) (-19.8255, -21.0154) (-19.8692, -21.1353) knots 0 0 0 0 1 1 1 1
  spline S1728 degree 3 poles (-19.8692, -21.1353) (-19.8569, -21.3462) (-19.8126, -21.5118) (-19.6806, -21.679) knots 0 0 0 0 1 1 1 1
  spline S1729 degree 3 poles (-19.6806, -21.679) (-19.4931, -21.8319) (-19.2458, -21.9006) (-19.0187, -21.9767) knots 0 0 0 0 1 1 1 1
  spline S1730 degree 3 poles (-19.0187, -21.9767) (-19.1249, -22.051) (-19.1249, -22.051) (-19.2229, -22.0137) knots 0 0 0 0 1 1 1 1
  spline S1731 degree 3 poles (-19.2229, -22.0137) (-19.827, -21.7553) (-20.4117, -21.4516) (-20.9532, -21.0786) knots 0 0 0 0 1 1 1 1
  spline S1732 degree 3 poles (-20.9532, -21.0786) (-20.9878, -21.0548) (-21.0224, -21.0311) (-21.0581, -21.0066) knots 0 0 0 0 1 1 1 1
  spline S1733 degree 3 poles (-21.0581, -21.0066) (-21.5152, -20.6695) (-21.7949, -20.25) (-22.0012, -19.7319) knots 0 0 0 0 1 1 1 1
  spline S1734 degree 3 poles (-22.0012, -19.7319) (-22.0572, -19.5919) (-22.1164, -19.4533) (-22.1756, -19.3146) knots 0 0 0 0 1 1 1 1
  spline S1735 degree 3 poles (-22.1756, -19.3146) (-22.1871, -19.2875) (-22.1986, -19.2605) (-22.2105, -19.2326) knots 0 0 0 0 1 1 1 1
  spline S1736 degree 3 poles (-22.2105, -19.2326) (-22.5108, -18.5323) (-22.9082, -17.9491) (-23.5944, -17.5788) knots 0 0 0 0 1 1 1 1
  spline S1737 degree 3 poles (-23.5944, -17.5788) (-23.8677, -17.5313) (-24.0813, -17.5542) (-24.3398, -17.656) knots 0 0 0 0 1 1 1 1
  spline S1738 degree 3 poles (-24.3398, -17.656) (-24.4357, -17.7272) (-24.4357, -17.7272) (-24.471, -17.8341) knots 0 0 0 0 1 1 1 1
  spline S1739 degree 3 poles (-24.471, -17.8341) (-24.4742, -17.8696) (-24.4773, -17.905) (-24.4805, -17.9416) knots 0 0 0 0 1 1 1 1
  spline S1740 degree 3 poles (-24.4805, -17.9416) (-24.4867, -17.9836) (-24.4929, -18.0256) (-24.4993, -18.0689) knots 0 0 0 0 1 1 1 1
  spline S1741 degree 3 poles (-24.4993, -18.0689) (-24.4721, -18.6096) (-24.0688, -18.9799) (-23.6983, -19.332) knots 0 0 0 0 1 1 1 1
  spline S1742 degree 3 poles (-23.6983, -19.332) (-23.6186, -19.4021) (-23.5376, -19.4698) (-23.4556, -19.5371) knots 0 0 0 0 1 1 1 1
  spline S1743 degree 3 poles (-23.4556, -19.5371) (-23.4642, -19.5659) (-23.4727, -19.5946) (-23.4816, -19.6243) knots 0 0 0 0 1 1 1 1
  spline S1744 degree 3 poles (-23.4816, -19.6243) (-24.3347, -19.4657) (-25.0612, -19.192) (-25.7908, -18.7096) knots 0 0 0 0 1 1 1 1
  spline S1745 degree 3 poles (-25.7908, -18.7096) (-25.8344, -18.6814) (-25.878, -18.6531) (-25.9229, -18.624) knots 0 0 0 0 1 1 1 1
  spline S1746 degree 3 poles (-25.9229, -18.624) (-26.4431, -18.279) (-26.8846, -17.8478) (-27.3154, -17.3985) knots 0 0 0 0 1 1 1 1
  spline S1747 degree 3 poles (-27.3154, -17.3985) (-27.3534, -17.3589) (-27.3534, -17.3589) (-27.3922, -17.3186) knots 0 0 0 0 1 1 1 1
  spline S1748 degree 3 poles (-27.3922, -17.3186) (-27.507, -17.1975) (-27.617, -17.0757) (-27.719, -16.9435) knots 0 0 0 0 1 1 1 1
  spline S1749 degree 3 poles (-27.719, -16.9435) (-27.9459, -16.6516) (-27.9459, -16.6516) (-28.1225, -16.583) knots 0 0 0 0 1 1 1 1
  spline S1750 degree 3 poles (-28.1225, -16.583) (-28.294, -16.5729) (-28.4039, -16.6105) (-28.5369, -16.7212) knots 0 0 0 0 1 1 1 1
  spline S1751 degree 3 poles (-28.5369, -16.7212) (-28.7119, -16.8875) (-28.8669, -17.07) (-29.0214, -17.2552) knots 0 0 0 0 1 1 1 1
  spline S1752 degree 3 poles (-29.0214, -17.2552) (-29.1123, -17.3707) (-29.1123, -17.3707) (-29.2405, -17.4178) knots 0 0 0 0 1 1 1 1
  spline S1753 degree 3 poles (-29.2405, -17.4178) (-28.9804, -17.6528) (-28.7121, -17.8757) (-28.4388, -18.0952) knots 0 0 0 0 1 1 1 1
  spline S1754 degree 3 poles (-28.4388, -18.0952) (-28.3131, -18.1963) (-28.1896, -18.2971) (-28.0742, -18.41) knots 0 0 0 0 1 1 1 1
  spline S1755 degree 3 poles (-28.0742, -18.41) (-28.3774, -18.4392) (-28.683, -18.3521) (-28.9291, -18.1735) knots 0 0 0 0 1 1 1 1
  spline S1756 degree 3 poles (-28.9291, -18.1735) (-29.3019, -17.8426) (-29.5348, -17.372) (-29.7757, -16.9434) knots 0 0 0 0 1 1 1 1
  spline S1757 degree 3 poles (-29.7757, -16.9434) (-29.9345, -16.6647) (-30.1137, -16.4101) (-30.3108, -16.1575) knots 0 0 0 0 1 1 1 1
  spline S1758 degree 3 poles (-30.3108, -16.1575) (-30.3946, -16.0618) (-30.3946, -16.0618) (-30.4044, -15.9707) knots 0 0 0 0 1 1 1 1
  spline S1759 degree 3 poles (-30.4044, -15.9707) (-30.4339, -15.9675) (-30.4633, -15.9642) (-30.4937, -15.9608) knots 0 0 0 0 1 1 1 1
  spline S1760 degree 3 poles (-30.4937, -15.9608) (-30.532, -15.9564) (-30.5704, -15.9521) (-30.6099, -15.9476) knots 0 0 0 0 1 1 1 1
  spline S1761 degree 3 poles (-30.6099, -15.9476) (-30.648, -15.9433) (-30.6862, -15.939) (-30.7255, -15.9346) knots 0 0 0 0 1 1 1 1
  spline S1762 degree 3 poles (-30.7255, -15.9346) (-30.825, -15.924) (-30.825, -15.924) (-30.9134, -15.8953) knots 0 0 0 0 1 1 1 1
  spline S1763 degree 3 poles (-30.9134, -15.8953) (-31.182, -15.909) (-31.3357, -15.9813) (-31.5262, -16.1685) knots 0 0 0 0 1 1 1 1
  spline S1764 degree 3 poles (-31.5262, -16.1685) (-31.5902, -16.26) (-31.5436, -16.3977) (-31.5318, -16.5026) knots 0 0 0 0 1 1 1 1
  spline S1765 degree 3 poles (-31.5318, -16.5026) (-31.5261, -16.5548) (-31.5203, -16.6071) (-31.5144, -16.661) knots 0 0 0 0 1 1 1 1
  spline S1766 degree 3 poles (-31.5144, -16.661) (-31.5097, -16.7015) (-31.5051, -16.7419) (-31.5003, -16.7836) knots 0 0 0 0 1 1 1 1
  spline S1767 degree 3 poles (-31.5003, -16.7836) (-31.4649, -16.7916) (-31.4649, -16.7916) (-31.4287, -16.7998) knots 0 0 0 0 1 1 1 1
  spline S1768 degree 3 poles (-31.4287, -16.7998) (-31.2972, -16.8454) (-31.1933, -16.9144) (-31.0766, -16.9903) knots 0 0 0 0 1 1 1 1
  spline S1769 degree 3 poles (-31.0766, -16.9903) (-30.8998, -17.1041) (-30.7229, -17.2142) (-30.539, -17.3163) knots 0 0 0 0 1 1 1 1
  spline S1770 degree 3 poles (-30.539, -17.3163) (-30.8479, -17.4835) (-31.3714, -17.3566) (-31.7031, -17.2737) knots 0 0 0 0 1 1 1 1
  spline S1771 degree 3 poles (-31.7031, -17.2737) (-32.2555, -17.1066) (-32.5731, -16.8305) (-32.8467, -16.3262) knots 0 0 0 0 1 1 1 1
  spline S1772 degree 3 poles (-32.8467, -16.3262) (-32.8748, -16.2736) (-32.9028, -16.221) (-32.9306, -16.1683) knots 0 0 0 0 1 1 1 1
  spline S1773 degree 3 poles (-32.9306, -16.1683) (-32.9618, -16.1749) (-32.993, -16.1815) (-33.0252, -16.1883) knots 0 0 0 0 1 1 1 1
  spline S1774 degree 3 poles (-33.0252, -16.1883) (-33.7379, -16.3352) (-34.3997, -16.4122) (-35.1293, -16.3495) knots 0 0 0 0 1 1 1 1
  spline S1775 degree 3 poles (-35.1293, -16.3495) (-35.1981, -16.3437) (-35.1981, -16.3437) (-35.2683, -16.3378) knots 0 0 0 0 1 1 1 1
  spline S1776 degree 3 poles (-35.2683, -16.3378) (-35.4551, -16.3219) (-35.6419, -16.3058) (-35.8285, -16.2869) knots 0 0 0 0 1 1 1 1
  spline S1777 degree 3 poles (-35.8285, -16.2869) (-36.434, -16.2266) (-36.9683, -16.2425) (-37.5624, -16.3577) knots 0 0 0 0 1 1 1 1
  spline S1778 degree 3 poles (-37.5624, -16.3577) (-37.6252, -16.3694) (-37.6879, -16.381) (-37.7507, -16.3926) knots 0 0 0 0 1 1 1 1
  spline S1779 degree 3 poles (-37.7507, -16.3926) (-37.9021, -16.4206) (-38.0534, -16.4494) (-38.2045, -16.4787) knots 0 0 0 0 1 1 1 1
  spline S1780 degree 3 poles (-38.2045, -16.4787) (-38.2092, -16.4522) (-38.2139, -16.4258) (-38.2187, -16.3985) knots 0 0 0 0 1 1 1 1
  spline S1781 degree 3 poles (-38.2187, -16.3985) (-38.1907, -16.3891) (-38.1627, -16.3796) (-38.1339, -16.3699) knots 0 0 0 0 1 1 1 1
  spline S1782 degree 3 poles (-38.1339, -16.3699) (-38.0935, -16.3562) (-38.0532, -16.3425) (-38.0116, -16.3285) knots 0 0 0 0 1 1 1 1
  spline S1783 degree 3 poles (-38.0116, -16.3285) (-37.965, -16.3127) (-37.9183, -16.2969) (-37.8703, -16.2806) knots 0 0 0 0 1 1 1 1
  spline S1784 degree 3 poles (-37.8703, -16.2806) (-37.7622, -16.2439) (-37.6544, -16.2065) (-37.5467, -16.1687) knots 0 0 0 0 1 1 1 1
  spline S1785 degree 3 poles (-37.5467, -16.1687) (-37.1557, -16.032) (-36.7627, -15.9053) (-36.366, -15.7864) knots 0 0 0 0 1 1 1 1
  spline S1786 degree 3 poles (-36.366, -15.7864) (-36.2543, -15.7527) (-36.143, -15.7177) (-36.0317, -15.6825) knots 0 0 0 0 1 1 1 1
  spline S1787 degree 3 poles (-36.0317, -15.6825) (-35.9744, -15.6653) (-35.9744, -15.6653) (-35.9159, -15.6479) knots 0 0 0 0 1 1 1 1
  spline S1788 degree 3 poles (-35.9159, -15.6479) (-35.6612, -15.5651) (-35.5433, -15.4919) (-35.4007, -15.264) knots 0 0 0 0 1 1 1 1
  spline S1789 degree 3 poles (-35.4007, -15.264) (-35.3858, -15.2411) (-35.3709, -15.2182) (-35.3556, -15.1946) knots 0 0 0 0 1 1 1 1
  spline S1790 degree 3 poles (-35.3556, -15.1946) (-35.2883, -15.0896) (-35.2335, -14.9863) (-35.1833, -14.8719) knots 0 0 0 0 1 1 1 1
  spline S1791 degree 3 poles (-35.1833, -14.8719) (-35.2545, -14.6242) (-35.3964, -14.4148) (-35.5838, -14.2403) knots 0 0 0 0 1 1 1 1
  spline S1792 degree 3 poles (-35.5838, -14.2403) (-35.8066, -14.1315) (-36.0398, -14.0845) (-36.2813, -14.0329) knots 0 0 0 0 1 1 1 1
  spline S1793 degree 3 poles (-36.2813, -14.0329) (-36.3792, -14.0111) (-36.477, -13.9892) (-36.5749, -13.9673) knots 0 0 0 0 1 1 1 1
  spline S1794 degree 3 poles (-36.5749, -13.9673) (-36.7366, -13.9314) (-36.8984, -13.8957) (-37.0603, -13.8605) knots 0 0 0 0 1 1 1 1
  spline S1795 degree 3 poles (-37.0603, -13.8605) (-38.4243, -13.5864) (-38.4243, -13.5864) (-39.4836, -12.7387) knots 0 0 0 0 1 1 1 1
  spline S1796 degree 3 poles (-39.4836, -12.7387) (-39.4883, -12.7123) (-39.4929, -12.6858) (-39.4977, -12.6586) knots 0 0 0 0 1 1 1 1
  spline S1797 degree 3 poles (-39.4977, -12.6586) (-39.8452, -12.5448) (-40.2666, -12.5203) (-40.6218, -12.6089) knots 0 0 0 0 1 1 1 1
  spline S1798 degree 3 poles (-40.6218, -12.6089) (-40.7861, -12.7141) (-40.8607, -12.8955) (-40.9198, -13.0768) knots 0 0 0 0 1 1 1 1
  spline S1799 degree 3 poles (-40.9198, -13.0768) (-40.9391, -13.1673) (-40.9417, -13.2493) (-40.9418, -13.3418) knots 0 0 0 0 1 1 1 1
  spline S1800 degree 3 poles (-40.9418, -13.3418) (-40.9448, -13.5631) (-41.0221, -13.7472) (-41.131, -13.9379) knots 0 0 0 0 1 1 1 1
  spline S1801 degree 3 poles (-41.131, -13.9379) (-41.2341, -14.0365) (-41.2799, -14.0615) (-41.4098, -14.1052) knots 0 0 0 0 1 1 1 1
  spline S1802 degree 3 poles (-41.4098, -14.1052) (-41.444, -14.1171) (-41.4781, -14.1291) (-41.5133, -14.1414) knots 0 0 0 0 1 1 1 1
  spline S1803 degree 3 poles (-41.5133, -14.1414) (-41.5494, -14.154) (-41.5855, -14.1666) (-41.6228, -14.1796) knots 0 0 0 0 1 1 1 1
  spline S1804 degree 3 poles (-41.6228, -14.1796) (-42.0028, -14.3184) (-42.3455, -14.4589) (-42.5783, -14.8076) knots 0 0 0 0 1 1 1 1
  spline S1805 degree 3 poles (-42.5783, -14.8076) (-42.6132, -14.9748) (-42.6179, -15.1056) (-42.5498, -15.2621) knots 0 0 0 0 1 1 1 1
  spline S1806 degree 3 poles (-42.5498, -15.2621) (-42.3631, -15.5124) (-42.1045, -15.7202) (-41.845, -15.8917) knots 0 0 0 0 1 1 1 1
  spline S1807 degree 3 poles (-41.845, -15.8917) (-41.7541, -15.9466) (-41.7541, -15.9466) (-41.7463, -16.0705) knots 0 0 0 0 1 1 1 1
  spline S1808 degree 3 poles (-41.7463, -16.0705) (-42.3437, -16.1996) (-42.9881, -16.1123) (-43.5537, -15.8935) knots 0 0 0 0 1 1 1 1
  spline S1809 degree 3 poles (-43.5537, -15.8935) (-43.6018, -15.8759) (-43.6498, -15.8584) (-43.6993, -15.8403) knots 0 0 0 0 1 1 1 1
  spline S1810 degree 3 poles (-43.6993, -15.8403) (-43.8876, -15.7657) (-43.8876, -15.7657) (-44.0509, -15.6507) knots 0 0 0 0 1 1 1 1
  spline S1811 degree 3 poles (-44.0509, -15.6507) (-44.1497, -15.3982) (-44.1079, -15.1366) (-44.0661, -14.8763) knots 0 0 0 0 1 1 1 1
  spline S1812 degree 3 poles (-44.0661, -14.8763) (-44.0557, -14.8062) (-44.0453, -14.7361) (-44.0349, -14.666) knots 0 0 0 0 1 1 1 1
  spline S1813 degree 3 poles (-44.0349, -14.666) (-44.0302, -14.6356) (-44.0254, -14.6051) (-44.0204, -14.5736) knots 0 0 0 0 1 1 1 1
  spline S1814 degree 3 poles (-44.0204, -14.5736) (-43.9954, -14.3937) (-44.0045, -14.248) (-44.0382, -14.0685) knots 0 0 0 0 1 1 1 1
  spline S1815 degree 3 poles (-44.0382, -14.0685) (-44.0461, -14.0254) (-44.0541, -13.9823) (-44.0623, -13.9378) knots 0 0 0 0 1 1 1 1
  spline S1816 degree 3 poles (-44.0623, -13.9378) (-44.0686, -13.9051) (-44.0749, -13.8723) (-44.0813, -13.8386) knots 0 0 0 0 1 1 1 1
  spline S1817 degree 3 poles (-44.0813, -13.8386) (-44.3004, -13.7449) (-44.4342, -13.7038) (-44.6704, -13.7772) knots 0 0 0 0 1 1 1 1
  spline S1818 degree 3 poles (-44.6704, -13.7772) (-44.7015, -13.804) (-44.7325, -13.8308) (-44.7645, -13.8583) knots 0 0 0 0 1 1 1 1
  spline S1819 degree 3 poles (-44.7645, -13.8583) (-45.0252, -14.028) (-45.3765, -13.9913) (-45.6795, -13.999) knots 0 0 0 0 1 1 1 1
  spline S1820 degree 3 poles (-45.6795, -13.999) (-45.9358, -14.0059) (-46.1902, -14.0242) (-46.4456, -14.0463) knots 0 0 0 0 1 1 1 1
  spline S1821 degree 3 poles (-46.4456, -14.0463) (-46.4812, -14.0493) (-46.5168, -14.0523) (-46.5535, -14.0554) knots 0 0 0 0 1 1 1 1
  spline S1822 degree 3 poles (-46.5535, -14.0554) (-46.6785, -14.0667) (-46.8032, -14.0795) (-46.928, -14.0927) knots 0 0 0 0 1 1 1 1
  spline S1823 degree 3 poles (-46.928, -14.0927) (-46.9783, -14.0979) (-47.0286, -14.1032) (-47.0805, -14.1087) knots 0 0 0 0 1 1 1 1
  spline S1824 degree 3 poles (-47.0805, -14.1087) (-47.7114, -14.1797) (-48.3348, -14.2952) (-48.9593, -14.4077) knots 0 0 0 0 1 1 1 1
  spline S1825 degree 3 poles (-48.9593, -14.4077) (-49.1646, -14.4447) (-49.37, -14.4813) (-49.5753, -14.5178) knots 0 0 0 0 1 1 1 1
  spline S1826 degree 3 poles (-49.5753, -14.5178) (-50.1587, -14.6216) (-50.742, -14.726) (-51.3252, -14.8307) knots 0 0 0 0 1 1 1 1
  spline S1827 degree 3 poles (-51.3252, -14.8307) (-51.6487, -14.8887) (-51.9722, -14.9465) (-52.2958, -15.0039) knots 0 0 0 0 1 1 1 1
  spline S1828 degree 3 poles (-52.2958, -15.0039) (-52.4658, -15.0341) (-52.6357, -15.0645) (-52.8056, -15.0952) knots 0 0 0 0 1 1 1 1
  spline S1829 degree 3 poles (-52.8056, -15.0952) (-53.9304, -15.2986) (-55.061, -15.4742) (-56.2046, -15.5244) knots 0 0 0 0 1 1 1 1
  spline S1830 degree 3 poles (-56.2046, -15.5244) (-56.2575, -15.5273) (-56.3105, -15.5302) (-56.3651, -15.5331) knots 0 0 0 0 1 1 1 1
  spline S1831 degree 3 poles (-56.3651, -15.5331) (-57.1638, -15.5727) (-57.9046, -15.4951) (-58.6805, -15.3026) knots 0 0 0 0 1 1 1 1
  spline S1832 degree 3 poles (-58.6805, -15.3026) (-59.009, -15.2218) (-59.2889, -15.1844) (-59.6222, -15.2493) knots 0 0 0 0 1 1 1 1
  spline S1833 degree 3 poles (-59.6222, -15.2493) (-59.6505, -15.2543) (-59.6788, -15.2593) (-59.7079, -15.2645) knots 0 0 0 0 1 1 1 1
  spline S1834 degree 3 poles (-59.7079, -15.2645) (-59.8331, -15.2876) (-59.9318, -15.3118) (-60.0445, -15.3728) knots 0 0 0 0 1 1 1 1
  spline S1835 degree 3 poles (-60.0445, -15.3728) (-60.2582, -15.4256) (-60.4204, -15.4148) (-60.6355, -15.3737) knots 0 0 0 0 1 1 1 1
  spline S1836 degree 3 poles (-60.6355, -15.3737) (-60.8943, -15.3294) (-61.1088, -15.325) (-61.3618, -15.3985) knots 0 0 0 0 1 1 1 1
  spline S1837 degree 3 poles (-61.3618, -15.3985) (-61.3927, -15.4073) (-61.4237, -15.416) (-61.4557, -15.4251) knots 0 0 0 0 1 1 1 1
  spline S1838 degree 3 poles (-61.4557, -15.4251) (-61.5293, -15.447) (-61.6023, -15.4708) (-61.6752, -15.4951) knots 0 0 0 0 1 1 1 1
  spline S1839 degree 3 poles (-61.6752, -15.4951) (-61.4084, -15.9903) (-61.4084, -15.9903) (-61.2318, -16.0623) knots 0 0 0 0 1 1 1 1
  spline S1840 degree 3 poles (-61.2318, -16.0623) (-61.1036, -16.124) (-61.1036, -16.124) (-61.0724, -16.2233) knots 0 0 0 0 1 1 1 1
  spline S1841 degree 3 poles (-61.0724, -16.2233) (-60.96, -16.7672) (-61.0326, -17.381) (-61.1288, -17.9232) knots 0 0 0 0 1 1 1 1
  spline S1842 degree 3 poles (-61.1288, -17.9232) (-61.1428, -18.0432) (-61.1365, -18.1145) (-61.1003, -18.2284) knots 0 0 0 0 1 1 1 1
  spline S1843 degree 3 poles (-61.1003, -18.2284) (-61.0872, -18.2716) (-61.0872, -18.2716) (-61.0739, -18.3157) knots 0 0 0 0 1 1 1 1
  spline S1844 degree 3 poles (-61.0739, -18.3157) (-61.037, -18.404) (-60.9881, -18.4682) (-60.9309, -18.5445) knots 0 0 0 0 1 1 1 1
  spline S1845 degree 3 poles (-60.9309, -18.5445) (-60.8773, -18.7158) (-60.8675, -18.7942) (-60.9427, -18.9593) knots 0 0 0 0 1 1 1 1
  spline S1846 degree 3 poles (-60.9427, -18.9593) (-61.0386, -19.1174) (-61.1649, -19.2025) (-61.3159, -19.3043) knots 0 0 0 0 1 1 1 1
  spline S1847 degree 3 poles (-61.3159, -19.3043) (-61.4961, -19.4347) (-61.6154, -19.5272) (-61.6624, -19.7552) knots 0 0 0 0 1 1 1 1
  spline S1848 degree 3 poles (-61.6624, -19.7552) (-61.6726, -19.8575) (-61.6734, -19.9569) (-61.6734, -20.0597) knots 0 0 0 0 1 1 1 1
  spline S1849 degree 3 poles (-61.6734, -20.0597) (-61.6784, -20.1677) (-61.7002, -20.2589) (-61.7281, -20.3632) knots 0 0 0 0 1 1 1 1
  spline S1850 degree 3 poles (-61.7281, -20.3632) (-61.7795, -20.5977) (-61.7623, -20.8041) (-61.6901, -21.0329) knots 0 0 0 0 1 1 1 1
  spline S1851 degree 3 poles (-61.6901, -21.0329) (-61.6697, -21.0644) (-61.6494, -21.0959) (-61.6284, -21.1283) knots 0 0 0 0 1 1 1 1
  spline S1852 degree 3 poles (-61.6284, -21.1283) (-61.5693, -21.2141) (-61.5693, -21.2141) (-61.5645, -21.3057) knots 0 0 0 0 1 1 1 1
  spline S1853 degree 3 poles (-61.5645, -21.3057) (-61.5939, -21.4137) (-61.6426, -21.4523) (-61.7273, -21.5248) knots 0 0 0 0 1 1 1 1
  spline S1854 degree 3 poles (-61.7273, -21.5248) (-62.1034, -21.8682) (-62.3805, -22.2895) (-62.5646, -22.7645) knots 0 0 0 0 1 1 1 1
  spline S1855 degree 3 poles (-62.5646, -22.7645) (-62.6295, -22.9065) (-62.6295, -22.9065) (-62.7705, -22.9307) knots 0 0 0 0 1 1 1 1
  spline S1856 degree 3 poles (-62.7705, -22.9307) (-63.0303, -22.9665) (-63.2925, -22.9572) (-63.5539, -22.9518) knots 0 0 0 0 1 1 1 1
  spline S1857 degree 3 poles (-63.5539, -22.9518) (-63.6316, -22.952) (-63.6316, -22.952) (-63.7109, -22.9521) knots 0 0 0 0 1 1 1 1
  spline S1858 degree 3 poles (-63.7109, -22.9521) (-64.0379, -22.9452) (-64.2619, -22.8885) (-64.5482, -22.7317) knots 0 0 0 0 1 1 1 1
  spline S1859 degree 3 poles (-64.5482, -22.7317) (-64.7229, -22.6427) (-64.9007, -22.6078) (-65.0924, -22.5725) knots 0 0 0 0 1 1 1 1
  spline S1860 degree 3 poles (-65.0924, -22.5725) (-65.3838, -22.5171) (-65.5922, -22.4689) (-65.7811, -22.2241) knots 0 0 0 0 1 1 1 1
  spline S1861 degree 3 poles (-65.7811, -22.2241) (-65.8801, -22.1021) (-65.8801, -22.1021) (-65.9744, -22.0361) knots 0 0 0 0 1 1 1 1
  spline S1862 degree 3 poles (-65.9744, -22.0361) (-66.0028, -21.9138) (-66.0028, -21.9138) (-66.0167, -21.7958) knots 0 0 0 0 1 1 1 1
  spline S1863 degree 3 poles (-66.0167, -21.7958) (-66.0494, -21.8) (-66.082, -21.8042) (-66.1157, -21.8085) knots 0 0 0 0 1 1 1 1
  spline S1864 degree 3 poles (-66.1157, -21.8085) (-66.1589, -21.8134) (-66.2022, -21.8184) (-66.2468, -21.8234) knots 0 0 0 0 1 1 1 1
  spline S1865 degree 3 poles (-66.2468, -21.8234) (-66.3108, -21.8311) (-66.3108, -21.8311) (-66.3762, -21.839) knots 0 0 0 0 1 1 1 1
  spline S1866 degree 3 poles (-66.3762, -21.839) (-66.554, -21.841) (-66.6702, -21.8025) (-66.8065, -21.688) knots 0 0 0 0 1 1 1 1
  spline S1867 degree 3 poles (-66.8065, -21.688) (-67.0567, -21.4143) (-67.268, -21.1231) (-67.4706, -20.8129) knots 0 0 0 0 1 1 1 1
  spline S1868 degree 3 poles (-67.4706, -20.8129) (-67.489, -20.7848) (-67.5074, -20.7567) (-67.5264, -20.7278) knots 0 0 0 0 1 1 1 1
  spline S1869 degree 3 poles (-67.5264, -20.7278) (-67.7332, -20.3771) (-67.8001, -19.9646) (-67.868, -19.5689) knots 0 0 0 0 1 1 1 1
  spline S1870 degree 3 poles (-67.868, -19.5689) (-67.8726, -19.5423) (-67.8772, -19.5158) (-67.8819, -19.4884) knots 0 0 0 0 1 1 1 1
  spline S1871 degree 3 poles (-67.8819, -19.4884) (-67.9831, -18.8943) (-67.9694, -18.3842) (-67.8591, -17.7926) knots 0 0 0 0 1 1 1 1
  spline S1872 degree 3 poles (-67.8591, -17.7926) (-67.8198, -17.5785) (-67.8042, -17.3793) (-67.8132, -17.1615) knots 0 0 0 0 1 1 1 1
  spline S1873 degree 3 poles (-67.8132, -17.1615) (-67.7959, -17.0427) (-67.7493, -17.0008) (-67.6609, -16.9223) knots 0 0 0 0 1 1 1 1
  spline S1874 degree 3 poles (-67.6609, -16.9223) (-67.607, -16.8854) (-67.5521, -16.8499) (-67.4964, -16.8158) knots 0 0 0 0 1 1 1 1
  spline S1875 degree 3 poles (-67.4964, -16.8158) (-67.3257, -16.7025) (-67.1914, -16.5901) (-67.1456, -16.3803) knots 0 0 0 0 1 1 1 1
  spline S1876 degree 3 poles (-67.1456, -16.3803) (-67.1364, -16.3217) (-67.1275, -16.2631) (-67.119, -16.2044) knots 0 0 0 0 1 1 1 1
  spline S1877 degree 3 poles (-67.119, -16.2044) (-67.0831, -16.0477) (-66.9894, -15.926) (-66.8619, -15.8313) knots 0 0 0 0 1 1 1 1
  spline S1878 degree 3 poles (-66.8619, -15.8313) (-66.7413, -15.809) (-66.6211, -15.7891) (-66.4998, -15.7707) knots 0 0 0 0 1 1 1 1
  spline S1879 degree 3 poles (-66.4998, -15.7707) (-66.4258, -15.7588) (-66.3517, -15.7468) (-66.2777, -15.7348) knots 0 0 0 0 1 1 1 1
  spline S1880 degree 3 poles (-66.2777, -15.7348) (-66.1607, -15.7159) (-66.0437, -15.6974) (-65.9265, -15.6797) knots 0 0 0 0 1 1 1 1
  spline S1881 degree 3 poles (-65.9265, -15.6797) (-65.8136, -15.6626) (-65.701, -15.6441) (-65.5883, -15.6255) knots 0 0 0 0 1 1 1 1